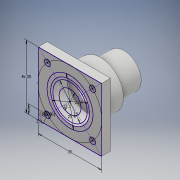
# Autodesk Inventor part: test de tolerancia
Saved by Autodesk Inventor 2018 (Build 220112000, 112)
## iProperties
Created: 2018-03-20
Part Number: test de tolerancia
Material: Generic
Document SubType Name: Modeling
Designer: Soichi
Density: 1 g/cm^3
Appearance: Default
Author: Soichi
Autodesk Inventor part; units mm, degrees
ref_plane "YZ Plane" through (0, 0, 0) normal (1, 0, 0) x (0, 1, 0)
ref_plane "XZ Plane" through (0, 0, 0) normal (0, 1, 0) x (-1, 0, 0)
ref_plane "XY Plane" through (0, 0, 0) normal (0, 0, 1) x (1, 0, 0)
sketch "Sketch1" plane through (0, 0, 0) normal (0, 1, 0) x (-1, 0, 0)
  line L0 (-17.5, 17.5) -> (17.5, 17.5)
  line L1 (17.5, 17.5) -> (17.5, -17.5)
  line L2 (17.5, -17.5) -> (-17.5, -17.5)
  line L3 (-17.5, -17.5) -> (-17.5, 17.5)
  line L4 (-17.5, 17.5) -> (17.5, -17.5) construction
  line L5 (17.5, 17.5) -> (-17.5, -17.5) construction
  circle A0 centre (12.5, -12.5) radius 1.65
  circle A1 centre (12.5, 12.5) radius 1.65
  circle A2 centre (-12.5, 12.5) radius 1.65
  circle A3 centre (-12.5, -12.5) radius 1.65
  circle A4 centre (0, 0) radius 6.05
  circle A5 centre (0, 0) radius 9.5
  circle A6 centre (0, 0) radius 12.7
  circle A7 centre (0, 0) radius 10.7
  dimension "d0" = 35
  dimension "d1" = 35
  dimension "d2" = 3.3
  dimension "d3" = 5
  dimension "d6" = 360
  dimension "d8" = 12.1
  dimension "d9" = 19
  dimension "d14" = 25.4
  dimension "d17" = 21.4
  constraints: 12 end point, 8 centre point, 4 coincident, 2 midpoint, 2 parallel, 1 horizontal, 1 perpendicular, 1 point on line, 9 other
  measures "d0" distance of L1.end L2.end
  measures "d1" distance of L0.end L1.end
  measures "d2" diameter of A0
  measures "d3" distance from line of L2 A0.centre
  measures "d8" diameter of A4
  measures "d9" diameter of A5
  measures "d14" diameter of A6
  measures "d17" diameter of A7
extrude "Extrusion1" add sketch "Sketch1" along normal blind 5 contours L0 L1 L2 L3 | A6
extrude "Extrusion2" add sketch "Sketch1" along normal blind 30 contours A5
extrude "Extrusion3" add sketch "Sketch1" along normal blind 17 contours A6 | A7
extrude "Extrusion4" cut sketch "Sketch1" along normal blind 10 contours A5 | A7
equation "\"d1\" = d0"
body "Solid1"
